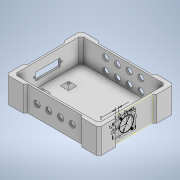
# Autodesk Inventor part: Case
Saved by Autodesk Inventor 2020 (Build 240168000, 168)
## iProperties
Created: 2020-06-02
Part Number: Case
Material: Generic
Document SubType Name: Modeling
Designer: Alex
Density: 1 g/cm^3
Appearance: Default
Author: Alex
Autodesk Inventor part; units mm, degrees
ref_plane "YZ Plane" through (0, 0, 0) normal (1, 0, 0) x (0, 1, 0)
ref_plane "XZ Plane" through (0, 0, 0) normal (0, 1, 0) x (-1, 0, 0)
ref_plane "XY Plane" through (0, 0, 0) normal (0, 0, 1) x (1, 0, 0)
sketch "Sketch1" plane through (0, 0, 0) normal (0, 1, 0) x (-1, 0, 0)
  line L0 (46, -60) -> (-46, -60)
  line L1 (-46, -60) -> (-50, -64)
  line L2 (-50, -64) -> (-75, -64)
  line L3 (-75, -64) -> (-79, -60)
  line L4 (-79, -60) -> (-79, -35)
  line L5 (-79, -35) -> (-75, -31)
  line L6 (-75, -31) -> (-75, 31)
  line L7 (-75, 31) -> (-79, 35)
  line L8 (-79, 35) -> (-79, 60)
  line L9 (-79, 60) -> (-75, 64)
  line L10 (-75, 64) -> (-50, 64)
  line L11 (-50, 64) -> (-46, 60)
  line L12 (-46, 60) -> (46, 60)
  line L13 (46, 60) -> (50, 64)
  line L14 (50, 64) -> (75, 64)
  line L15 (75, 64) -> (79, 60)
  line L16 (79, 60) -> (79, 35)
  line L17 (79, 35) -> (75, 31)
  line L18 (75, 31) -> (75, -31)
  line L19 (75, -31) -> (79, -35)
  line L20 (79, -35) -> (79, -60)
  line L21 (79, -60) -> (75, -64)
  line L22 (75, -64) -> (50, -64)
  line L23 (50, -64) -> (46, -60)
  point P0 (0, 0)
  point P1 (0, -60)
  point P2 (0, 60)
  point P3 (75, 0)
  point P4 (-75, 0)
  dimension "d0" = 135
  dimension "d1" = 120
  dimension "d2" = 150
  dimension "d3" = 4
  dimension "d4" = 25
  constraints: 48 end point, 9 equal length, 9 parallel, 9 perpendicular, 6 point on line, 4 midpoint, 3 collinear, 3 horizontal alignment, 3 vertical alignment, 1 horizontal
  measures "d0" angle of L0 L23
  measures "d1" distance between parallel lines of L12 L0
  measures "d2" distance between parallel lines of L6 L18
  measures "d3" distance between parallel lines of L0 L2
  measures "d4" distance of L1.end L2.end
extrude "Extrusion1" add sketch "Sketch1" along normal blind 3
sketch "Sketch2" plane through (0, 3, 0) normal (0, 1, 0) x (1, 0, 0)
  line L0 (79, 60) -> (75, 64) projected
  line L1 (75, 64) -> (50, 64) projected
  line L2 (50, 64) -> (46, 60) projected
  line L3 (46, 60) -> (-46, 60) projected
  line L4 (-46, 60) -> (-50, 64) projected
  line L5 (-50, 64) -> (-75, 64) projected
  line L6 (-75, 64) -> (-79, 60) projected
  line L7 (-79, 60) -> (-79, 35) projected
  line L8 (-79, 35) -> (-75, 31) projected
  line L9 (-75, 31) -> (-75, -31) projected
  line L10 (-75, -31) -> (-79, -35) projected
  line L11 (-79, -35) -> (-79, -60) projected
  line L12 (-79, -60) -> (-75, -64) projected
  line L13 (-75, -64) -> (-50, -64) projected
  line L14 (-50, -64) -> (-46, -60) projected
  line L15 (-46, -60) -> (46, -60) projected
  line L16 (46, -60) -> (50, -64) projected
  line L17 (50, -64) -> (75, -64) projected
  line L18 (75, -64) -> (79, -60) projected
  line L19 (79, -60) -> (79, -35) projected
  line L20 (79, -35) -> (75, -31) projected
  line L21 (75, -31) -> (75, 31) projected
  line L22 (75, 31) -> (79, 35) projected
  line L23 (79, 35) -> (79, 60) projected
  line L24 (-47.2426, 57) -> (47.2426, 57)
  line L25 (47.2426, 57) -> (51.2426, 61) construction
  line L26 (51.2426, 61) -> (73.7574, 61) construction
  line L27 (73.7574, 61) -> (76, 58.7574) construction
  line L28 (76, 58.7574) -> (76, 36.2426) construction
  line L29 (76, 36.2426) -> (72, 32.2426) construction
  line L30 (72, 32.2426) -> (72, -32.2426)
  line L31 (72, -32.2426) -> (76, -36.2426) construction
  line L32 (76, -36.2426) -> (76, -58.7574) construction
  line L33 (76, -58.7574) -> (73.7574, -61) construction
  line L34 (73.7574, -61) -> (51.2426, -61) construction
  line L35 (51.2426, -61) -> (47.2426, -57) construction
  line L36 (47.2426, -57) -> (-47.2426, -57)
  line L37 (-47.2426, -57) -> (-51.2426, -61) construction
  line L38 (-51.2426, -61) -> (-73.7574, -61) construction
  line L39 (-73.7574, -61) -> (-76, -58.7574) construction
  line L40 (-76, -58.7574) -> (-76, -36.2426) construction
  line L41 (-76, -36.2426) -> (-72, -32.2426) construction
  line L42 (-72, -32.2426) -> (-72, 32.2426)
  line L43 (-72, 32.2426) -> (-76, 36.2426) construction
  line L44 (-76, 36.2426) -> (-76, 58.7574) construction
  line L45 (-76, 58.7574) -> (-73.7574, 61) construction
  line L46 (-73.7574, 61) -> (-51.2426, 61) construction
  line L47 (-51.2426, 61) -> (-47.2426, 57) construction
  line L48 (-47.2426, 57) -> (-68, 57)
  line L49 (-72, 53) -> (-72, 32.2426)
  line L50 (-72, -32.2426) -> (-72, -53)
  line L51 (-68, -57) -> (-47.2426, -57)
  line L52 (47.2426, -57) -> (68, -57)
  line L53 (72, -53) -> (72, -32.2426)
  line L54 (47.2426, 57) -> (68, 57)
  line L55 (72, 53) -> (72, 32.2426)
  line L56 (-72, 53) -> (-68, 57)
  line L57 (-72, -53) -> (-68, -57)
  line L58 (68, -57) -> (72, -53)
  line L59 (72, 53) -> (68, 57)
  point P0 (0, 0)
  point P1 (-72, 57)
  point P2 (-72, -57)
  point P3 (72, -57)
  point P4 (72, 57)
  dimension "d7" = 3
  dimension "d8" = 4
  dimension "d9" = 4
  dimension "d10" = 4
  dimension "d11" = 4
  dimension "d12" = 4
  dimension "d13" = 4
  dimension "d14" = 4
  dimension "d15" = 4
  constraints: 72 end point, 9 point on line, 4 horizontal, 2 perpendicular, 1 vertical, 23 other
  measures "d7" distance between parallel lines of L3 L24
  measures "d8" distance of L49.start point (-72, 57)
  measures "d9" distance of L48.end point (-72, 57)
  measures "d10" distance of L50.end point (-72, -57)
  measures "d11" distance of L51.start point (-72, -57)
  measures "d12" distance of L52.end point (72, -57)
  measures "d13" distance of L53.start point (72, -57)
  measures "d14" distance of L55.start point (72, 57)
  measures "d15" distance of L54.end point (72, 57)
extrude "Extrusion2" add sketch "Sketch2" along normal blind 40
sketch "Sketch3" plane through (0, 3, 0) normal (0, 1, 0) x (1, 0, 0)
  line L0 (63.5, -24) -> (-63.5, -24) construction
  line L1 (-63.5, -24) -> (-63.5, 24) construction
  line L2 (-63.5, 24) -> (63.5, 24) construction
  line L3 (63.5, 24) -> (63.5, -24) construction
  line L4 (63.5, -24) -> (-63.5, 24) construction
  line L5 (-63.5, -24) -> (63.5, 24) construction
  line L6 (-51.5, 15) -> (-45.5, 15)
  line L7 (-45.5, 15) -> (-45.5, 9)
  line L8 (-45.5, 9) -> (-51.5, 9)
  line L9 (-51.5, 9) -> (-51.5, 15)
  line L10 (-51.5, 15) -> (-45.5, 9) construction
  line L11 (-45.5, 15) -> (-51.5, 9) construction
  line L12 (-63.5, -24) -> (-57.5, -24)
  line L13 (-57.5, -24) -> (-57.5, -18)
  line L14 (-57.5, -18) -> (-63.5, -18)
  line L15 (-63.5, -18) -> (-63.5, -24)
  line L16 (-63.5, -24) -> (-57.5, -18) construction
  line L17 (-57.5, -24) -> (-63.5, -18) construction
  line L18 (39.5, -18) -> (45.5, -18)
  line L19 (45.5, -18) -> (45.5, -24)
  line L20 (45.5, -24) -> (39.5, -24)
  line L21 (39.5, -24) -> (39.5, -18)
  line L22 (39.5, -18) -> (45.5, -24) construction
  line L23 (45.5, -18) -> (39.5, -24) construction
  line L24 (57.5, 24) -> (63.5, 24)
  line L25 (63.5, 24) -> (63.5, 18)
  line L26 (63.5, 18) -> (57.5, 18)
  line L27 (57.5, 18) -> (57.5, 24)
  line L28 (57.5, 24) -> (63.5, 18) construction
  line L29 (63.5, 24) -> (57.5, 18) construction
  point P0 (0, 0)
  point P1 (-48.5, 12)
  point P2 (-60.5, -21)
  point P3 (42.5, -21)
  point P4 (60.5, 21)
  dimension "d18" = 127
  dimension "d19" = 48
  dimension "d20" = 12
  dimension "d21" = 15
  dimension "d22" = 3
  dimension "d23" = 3
  dimension "d24" = 3
  dimension "d25" = 3
  dimension "d26" = 21
  dimension "d27" = 3
  dimension "d28" = 6
  constraints: 60 end point, 10 midpoint, 10 parallel, 6 equal length, 5 horizontal, 5 perpendicular, 1 point on line
  measures "d18" distance of L1.end L2.end
  measures "d19" distance of L2.end L0.start
  measures "d20" distance from line of point (-48.5, 12) L2
  measures "d21" distance from line of point (-48.5, 12) L1
  measures "d22" distance from line of point (-60.5, -21) L0
  measures "d23" distance from line of point (-60.5, -21) L1
  measures "d24" distance from line of L3 point (60.5, 21)
  measures "d25" distance from line of L2 point (60.5, 21)
  measures "d26" distance from line of point (42.5, -21) L3
  measures "d27" distance from line of point (42.5, -21) L0
  measures "d28" distance of L6.end L7.end
extrude "Extrusion3" add sketch "Sketch3" along normal blind 4
chamfer "Chamfer1" distance 4 angle 45 16 edges at (42.5, 3, 24) (45.5, 3, 21) (60.5, 3, -18) (63.5, 3, -21) (39.5, 3, 21) (57.5, 3, -21) (42.5, 3, 18) (60.5, 3, -24) (-60.5, 3, 18) (-63.5, 3, 21) (-48.5, 3, -15) (-51.5, 3, -12) (-60.5, 3, 24) (-57.5, 3, 21) (-48.5, 3, -9) (-45.5, 3, -12)
sketch "Sketch4" plane through (-46, 0, 60) normal (0, 0, 1) x (1, 0, 0)
  line L0 (0, 0) -> (92, 0) construction
  line L1 (92, 0) -> (92, 43) construction
  line L2 (0, 43) -> (92, 43) construction
  line L3 (0, 0) -> (0, 43) construction
  line L4 (0, 0) -> (0, 43) construction
  line L5 (0, 43) -> (92, 43) construction
  line L6 (46, 43) -> (46, 0) construction
  point P0 (16, 21.5)
  point P1 (36, 21.5)
  point P2 (56, 21.5)
  point P3 (76, 21.5)
  point P4 (0, 21.5)
  dimension "d36" = 20
  constraints: 2 end point, 2 midpoint, 1 horizontal, 1 horizontal alignment, 1 perpendicular, 1 symmetric about line, 3 other
  measures "d36" distance of point (16, 21.5) point (36, 21.5)
hole "Hole1" at (-30, 21.5, 60) at (-10, 21.5, 60) at (10, 21.5, 60) at (30, 21.5, 60) direction (0, 0, -1) diameter 10.317 depth 3 clearance for "Hex Head Bolt" size "3/8" standard "Ansi Unified Screw Threads"
sketch "Sketch5" plane through (46, 0, -60) normal (0, 0, -1) x (-1, 0, 0)
  line L0 (0, 0) -> (92, 0) construction
  line L1 (92, 0) -> (92, 43) construction
  line L2 (0, 43) -> (92, 43) construction
  line L3 (0, 0) -> (0, 43) construction
  line L4 (0, 0) -> (0, 43) construction
  line L5 (0, 21.5) -> (92, 21.5) construction
  line L6 (92, 43) -> (0, 43) construction
  line L7 (46, 43) -> (46, 0) construction
  point P0 (16, 11.5)
  point P1 (36, 11.5)
  point P2 (56, 11.5)
  point P3 (76, 11.5)
  point P4 (16, 31.5)
  point P5 (36, 31.5)
  point P6 (56, 31.5)
  point P7 (76, 31.5)
  dimension "d50" = 20
  dimension "d53" = 20
  constraints: 4 end point, 3 midpoint, 2 symmetric about line, 2 vertical, 1 horizontal, 7 other
  measures "d50" distance of point (16, 11.5) point (36, 11.5)
  measures "d53" distance of point (16, 11.5) point (16, 31.5)
hole "Hole2" at (30, 11.5, -60) at (10, 11.5, -60) at (-10, 11.5, -60) at (-30, 11.5, -60) at (30, 31.5, -60) at (10, 31.5, -60) at (-10, 31.5, -60) at (-30, 31.5, -60) direction (0, 0, 1) diameter 10.317 depth 3 clearance for "Hex Head Bolt" size "3/8" standard "Ansi Unified Screw Threads"
sketch "Sketch6" plane through (0, 7, 0) normal (0, 1, 0) x (1, 0, 0)
  line L0 (45.5, -18) -> (39.5, -18) construction
  line L1 (39.5, -18) -> (39.5, -24) construction
  line L2 (39.5, -24) -> (45.5, -24) construction
  line L3 (45.5, -24) -> (45.5, -18) construction
  line L4 (63.5, 24) -> (57.5, 24) construction
  line L5 (57.5, 24) -> (57.5, 18) construction
  line L6 (57.5, 18) -> (63.5, 18) construction
  line L7 (63.5, 18) -> (63.5, 24) construction
  line L8 (-51.5, 9) -> (-45.5, 9) construction
  line L9 (-45.5, 9) -> (-45.5, 15) construction
  line L10 (-45.5, 15) -> (-51.5, 15) construction
  line L11 (-51.5, 15) -> (-51.5, 9) construction
  line L12 (-63.5, -18) -> (-63.5, -24) construction
  line L13 (-63.5, -24) -> (-57.5, -24) construction
  line L14 (-57.5, -24) -> (-57.5, -18) construction
  line L15 (-57.5, -18) -> (-63.5, -18) construction
  point P0 (0, 0)
  point P1 (42.5, -21)
  point P2 (60.5, 21)
  point P3 (-48.5, 12)
  point P4 (-60.5, -21)
  point P5 (39.5, -21)
  point P6 (-63.5, -21)
  point P7 (-51.5, 12)
  point P8 (57.5, 21)
  point P9 (42.5, -18)
  point P10 (60.5, 24)
  point P11 (-48.5, 15)
  point P12 (-60.5, -18)
  constraints: 8 midpoint, 4 horizontal alignment, 4 vertical alignment
hole "Hole3" at (42.5, 7, 21) at (60.5, 7, -21) at (-48.5, 7, -12) at (-60.5, 7, 21) direction (0, -1, 0) diameter 4 depth 5
sketch "Sketch7" plane through (-75, 0, -31) normal (-1, 0, 0) x (0, 0, 1)
  line L0 (52, 15) -> (10, 15)
  line L1 (10, 15) -> (10, 28)
  line L2 (10, 28) -> (52, 28)
  line L3 (52, 28) -> (52, 15)
  line L4 (52, 15) -> (10, 28) construction
  line L5 (10, 15) -> (52, 28) construction
  line L6 (0, 0) -> (62, 0) construction
  line L7 (62, 0) -> (62, 43) construction
  line L8 (0, 43) -> (62, 43) construction
  line L9 (0, 0) -> (0, 43) construction
  point P0 (31, 0)
  point P1 (31, 21.5)
  point P2 (31, 43)
  point P3 (31, 21.5)
  point P4 (10, 21.5)
  point P5 (0, 21.5)
  dimension "d70" = 42
  dimension "d71" = 13
  constraints: 12 end point, 6 midpoint, 2 parallel, 1 horizontal, 1 horizontal alignment, 1 perpendicular, 1 vertical alignment
  measures "d70" distance of L1.end L2.end
  measures "d71" distance of L2.end L0.start
extrude "Extrusion4" cut sketch "Sketch7" against normal up to surface (3 mm away)
sketch "Sketch8" plane through (-75, 0, -31) normal (-1, 0, 0) x (0, 0, 1)
  line L0 (4.5, 28) -> (57.5, 28) construction
  line L1 (57.5, 28) -> (57.5, 15) construction
  line L2 (57.5, 15) -> (4.5, 15) construction
  line L3 (4.5, 15) -> (4.5, 28) construction
  line L4 (10, 28) -> (52, 28) construction
  line L5 (52, 28) -> (52, 15) construction
  line L6 (52, 15) -> (10, 15) construction
  line L7 (10, 15) -> (10, 28) construction
  line L8 (0, 0) -> (62, 0) construction
  line L9 (62, 0) -> (62, 43) construction
  line L10 (0, 43) -> (62, 43) construction
  line L11 (0, 0) -> (0, 43) construction
  point P0 (31, 0)
  point P1 (31, 28)
  point P2 (31, 28)
  point P3 (10, 21.5)
  point P4 (4.5, 21.5)
  point P5 (7.5, 21.5)
  point P6 (54.5, 21.5)
  point P7 (52, 21.5)
  dimension "d75" = 53
  dimension "d76" = 3
  dimension "d77" = 3
  constraints: 8 end point, 5 midpoint, 3 horizontal alignment, 2 parallel, 1 coincident, 1 collinear, 1 horizontal, 1 perpendicular
  measures "d75" distance between parallel lines of L3 L1
  measures "d76" distance from line of L3 point (7.5, 21.5)
  measures "d77" distance from line of L1 point (54.5, 21.5)
hole "Hole4" at (-75, 21.5, -23.5) at (-75, 21.5, 23.5) direction (1, 0, 0) diameter 3 depth 3
sketch "Sketch9" plane through (75, 0, 31) normal (1, 0, 0) x (0, 0, -1)
  circle A0 centre (18, 21.5) radius 12
  circle A1 centre (8.5, 33.5) radius 1.75
  circle A2 centre (27.5, 9.5) radius 1.75
  line L0 (31, 6) -> (5, 6) construction
  line L1 (5, 6) -> (5, 37) construction
  line L2 (5, 37) -> (31, 37) construction
  line L3 (31, 37) -> (31, 6) construction
  line L4 (31, 6) -> (5, 37) construction
  line L5 (5, 6) -> (31, 37) construction
  line L6 (0, 0) -> (62, 0) construction
  line L7 (62, 0) -> (62, 43) construction
  line L8 (0, 43) -> (62, 43) construction
  line L9 (0, 0) -> (0, 43) construction
  point P0 (31, 0)
  point P1 (5, 21.5)
  point P2 (0, 21.5)
  dimension "d85" = 19
  dimension "d86" = 24
  dimension "d87" = 24
  dimension "d88" = 9.5
  dimension "d89" = 12
  dimension "d90" = 3.5
  dimension "d91" = 26
  dimension "d92" = 31
  dimension "d93" = 5
  constraints: 12 end point, 4 midpoint, 3 centre point, 2 parallel, 1 equal radius, 1 horizontal, 1 horizontal alignment, 1 perpendicular
  measures "d85" horizontal distance of A2.centre A1.centre
  measures "d86" vertical distance of A2.centre A1.centre
  measures "d87" diameter of A0
  measures "d88" horizontal distance of A0.centre A1.centre
  measures "d89" vertical distance of A0.centre A1.centre
  measures "d90" diameter of A1
  measures "d91" distance of L1.end L2.end
  measures "d92" distance of L2.end L0.start
  measures "d93" distance between parallel lines of L9 L1
equation "\"d9\" = d8"
equation "\"d10\" = d8"
equation "\"d11\" = d10"
equation "\"d12\" = d8"
equation "\"d13\" = d12"
equation "\"d14\" = d8"
equation "\"d15\" = d14"
equation "\"d77\" = d76"
equation "\"d88\" = 0.5 * d85"
equation "\"d89\" = 0.5 * d86"
body "Solid1"
